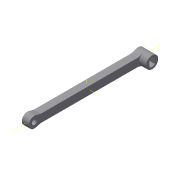
# Autodesk Inventor part: empty
Saved by Autodesk Inventor 2014 (Build 180170000, 170)
## iProperties
Created: 2015-04-13
Part Number: empty
Material: Generic
Document SubType Name: Modeling
Designer: Martin
Density: 1 g/cm^3
Appearance: Default
Author: Martin
Autodesk Inventor part; units mm, degrees
ref_plane "YZ Plane" through (0, 0, 0) normal (1, 0, 0) x (0, 1, 0)
ref_plane "XZ Plane" through (0, 0, 0) normal (0, 1, 0) x (-1, 0, 0)
ref_plane "XY Plane" through (0, 0, 0) normal (0, 0, 1) x (1, 0, 0)
sketch "Sketch1" plane through (0, 0, 0) normal (1, 0, 0) x (0, 1, 0)
  line L0 (-42.7, 0) -> (42.7, 0) projected
  line L1 (0, -4.2) -> (0, 4.2) projected
  circle A0 centre (-27.5, 0) radius 1.25
  circle A1 centre (-27.5, 0) radius 3
  circle A2 centre (27.5, 0) radius 3 construction
  line L2 (-27.5, 3) -> (27.5, 3)
  line L3 (-27.5, -3) -> (27.5, -3)
  line L4 (27.5, 3) -> (27.5, -3) construction
  line L5 (27.5, 2) -> (27.5, -2) construction
  arc A3 (27.5, -3) -> (27.5, 3) centre (27.5, 0) ccw
  circle A4 centre (-27.5, 0) radius 2.2678 construction
  circle A5 centre (27.5, 0) radius 1
  point P0 (0, 0)
  dimension "d4" = 6
  dimension "d7" = 55
  dimension "d8" = 2.5
  dimension "d10" = 0
  dimension "d30" = 2
  constraints: 8 end point, 6 centre point, 6 point on circle, 5 tangent, 3 coincident, 2 midpoint, 2 point on line, 1 equal radius, 1 parallel, 1 perpendicular, 1 symmetric about line
  measures "d4" diameter of A2
  measures "d7" distance of A2.centre A0.centre
  measures "d8" diameter of A0
  measures "d10" distance between parallel lines of L4 L5
  measures "d30" diameter of A5
extrude "ext_main" add sketch "Sketch1" along normal mid plane 3.5 contours A0 L0 A1 | L0 A1 A0 | A1 L2 L1 L0 | L0 L1 L3 A1 | L1 L2 A3 L0 A5 | L0 A5 A3 L3 L1
sketch "Sketch3" plane through (0, 0, 0) normal (1, 0, 0) x (0, 1, 0)
  arc A0 (-27.5, 3) -> (-27.5, -3) centre (-27.5, 0) ccw projected
  circle A1 centre (-27.5, 0) radius 1.25 projected
  arc A2 (27.5, -3) -> (27.5, 3) centre (27.5, 0) ccw projected
  circle A3 centre (-27.5, 0) radius 3 construction
  circle A4 centre (27.5, 0) radius 3 construction
  line L0 (-25.2639, 2) -> (25.2639, 2) construction
  line L1 (-42.7, 0) -> (42.7, 0) projected
  line L2 (0, -4.2579) -> (0, 4.2579) projected
  line L3 (27.5, 3) -> (-27.5, 3) projected
  line L4 (24.1192, 2) -> (26.5141, 2.8334)
  arc A5 (27.5, 3) -> (26.5141, 2.8334) centre (27.5, 0) ccw
  line L5 (-24.3389, 2) -> (24.1192, 2)
  circle A6 centre (-27.5, 0) radius 2.75
  line L6 (-24.3389, 2) -> (-26.7882, 2.6563)
  arc A7 (26.5141, -2.8334) -> (27.5, -3) centre (27.5, 0) ccw
  line L7 (24.1192, -2) -> (-25.2639, -2) construction
  line L8 (-24.3389, -2) -> (-26.7882, -2.6563)
  line L9 (24.1192, -2) -> (-24.3389, -2)
  line L10 (24.1192, -2) -> (26.5141, -2.8334)
  point P0 (0, 0)
  dimension "d16" = 1
  dimension "d21" = 5.5
  dimension "d22" = 15
  constraints: 16 end point, 11 point on circle, 5 centre point, 4 concentric, 3 coincident, 3 point on line, 2 parallel, 2 tangent, 1 collinear, 1 equal length, 3 other
  measures "d16" distance between parallel lines of L0 L3
  measures "d21" diameter of A6
  measures "d22" angle of L0 L6
extrude "ext_cutaway" cut sketch "Sketch3" along normal through all both and the other way through all contours A6 L1 A1 | L1 A1 A6 | L5 L4 A5 A2 L1 L2 | L2 L1 A6 L6 L5 | A6 L1 L2 L9 L8 | L1 A2 A7 L10 L9 L2 keep common part
sketch "Sketch4" plane through (1.75, 0, 0) normal (1, 0, 0) x (0, 0, -1)
  arc A0 (2.8334, 26.5141) -> (-2.8334, 26.5141) centre (0, 27.5) ccw projected
  circle A1 centre (0, 27.5) radius 1 projected
  circle A2 centre (0, 27.5) radius 3
  line L0 (-4.2, 0) -> (4.2, 0) projected
  line L1 (-3, 27.5) -> (3, 27.5) construction
  circle A3 centre (0, 27.5) radius 2 construction
  arc A4 (-1.4283, 28.9) -> (-1.4283, 26.1) centre (0, 27.5) ccw
  arc A5 (1.4283, 26.1) -> (1.4283, 28.9) centre (0, 27.5) ccw
  line L2 (-1.4283, 28.9) -> (1.4283, 28.9)
  line L3 (-1.4283, 26.1) -> (1.4283, 26.1)
  point P0 (0, 0)
  dimension "d23" = 4
  dimension "d25" = 2.8
  constraints: 9 point on circle, 6 end point, 4 centre point, 4 concentric, 3 coincident, 3 parallel, 1 midpoint, 1 other
  measures "d23" diameter of A3
  measures "d25" distance between parallel lines of L3 L2
extrude "ext_potshaft" add sketch "Sketch4" along normal blind 3.5 contours A2 A0
extrude "ext_cut_potshaft" cut sketch "Sketch4" against normal blind 1 contours L2 A5 L3 A4
equation "\"d8\" = screw_m2_bore_loose"
equation "\"d30\" = screw_m2_bore_selfthreading"
equation "\"d21\" = general_bore_smallersupport_diameter"
equation "\"screw_m2_bore_loose\" = 2.5"
equation "\"screw_m2_bore_selfthreading\" = 2"
equation "\"general_bore_smallersupport_diameter\" = 5.5"
body "Solid2"
